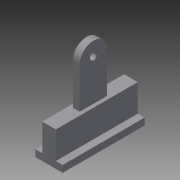
# Autodesk Inventor part: slider
Saved by Autodesk Inventor 2015 (Build 190159000, 159)
## iProperties
Created: 2015-04-09
Part Number: slider
Material: Generic
Document SubType Name: Modeling
Designer: WASHHSST
Density: 1 g/cm^3
Appearance: Default
Author: WASHHSST
Autodesk Inventor part; units mm, degrees
ref_plane "YZ Plane" through (0, 0, 0) normal (1, 0, 0) x (0, 1, 0)
ref_plane "XZ Plane" through (0, 0, 0) normal (0, 1, 0) x (-1, 0, 0)
ref_plane "XY Plane" through (0, 0, 0) normal (0, 0, 1) x (1, 0, 0)
sketch "Sketch1" plane through (0, 0, 0) normal (0, 0, 1) x (1, 0, 0)
  line L0 (0, 0) -> (25.4, 0)
  line L1 (25.4, 0) -> (25.4, 6.35)
  line L2 (25.4, 6.35) -> (19.05, 6.35)
  line L3 (19.05, 6.35) -> (19.05, 31.75)
  line L4 (19.05, 31.75) -> (6.35, 31.75)
  line L5 (6.35, 31.75) -> (6.35, 6.35)
  line L6 (6.35, 6.35) -> (0, 6.35)
  line L7 (0, 6.35) -> (0, 0)
  dimension "d0" = 12.7
  dimension "d1" = 6.35
  dimension "d2" = 6.35
  dimension "d3" = 6.35
  dimension "d4" = 25.4
  constraints: 16 end point, 6 perpendicular, 2 point on line, 1 horizontal
  measures "d0" distance between parallel lines of L3 L5
  measures "d1" distance between parallel lines of L0 L6
  measures "d2" distance from line of L6.end L5
  measures "d3" distance of L1.end L2.end
  measures "d4" distance between parallel lines of L6 L4
extrude "Extrusion1" add sketch "Sketch1" along normal blind 76.2
sketch "Sketch2" plane through (6.35, 31.75, 0) normal (0, 1, 0) x (1, 0, 0)
  line L0 (9.525, -50.8) -> (3.175, -50.8)
  line L1 (3.175, -50.8) -> (3.175, -25.4)
  line L2 (3.175, -25.4) -> (9.525, -25.4)
  line L3 (9.525, -25.4) -> (9.525, -50.8)
  line L4 (0, 0) -> (0, -76.2) projected
  line L5 (12.7, 0) -> (12.7, -76.2) projected
  line L6 (12.7, -76.2) -> (0, -76.2) projected
  line L7 (12.7, 0) -> (0, 0) projected
  point P0 (-6.35, 0)
  dimension "d7" = 12.7
  dimension "d8" = 3.175
  dimension "d9" = 3.175
  dimension "d10" = 6.35
  dimension "d11" = 76.2
  dimension "d12" = 25.4
  dimension "d13" = 25.4
  constraints: 8 end point, 2 parallel, 1 horizontal, 1 perpendicular
  measures "d7" distance between parallel lines of L4 L5
  measures "d8" distance between parallel lines of L3 L5
  measures "d9" distance between parallel lines of L4 L1
  measures "d10" distance between parallel lines of L1 L3
  measures "d11" distance between parallel lines of L6 L7
  measures "d12" distance between parallel lines of L6 L0
  measures "d13" distance between parallel lines of L0 L2
extrude "Extrusion2" add sketch "Sketch2" along normal blind 50.8 contours L0 L1 L2 L3
fillet "Fillet1" radius 12.7 2 edges at (12.7, 82.55, 50.8) (12.7, 82.55, 25.4)
hole "Hole1" at (15.875, 69.85, 38.1) direction (-1, 0, 0) diameter 6.35 end through all
body "Solid1"
